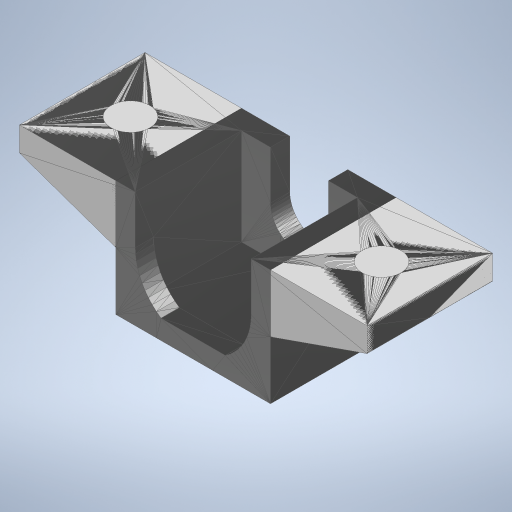
# Autodesk Inventor part: N20
Saved by Autodesk Inventor 2024 (Build 280153020, 153B)
## iProperties
Created: 2025-01-23
Part Number: N20
Material: Ogólny
Document SubType Name: Modeling
Designer: jakub
Density: 1 g/cm^3
Appearance: Domyślna
Author: jakub
Autodesk Inventor part; units mm, degrees
ref_plane "YZ Plane" through (0, 0, 0) normal (1, 0, 0) x (0, 1, 0)
ref_plane "XZ Plane" through (0, 0, 0) normal (0, 1, 0) x (-1, 0, 0)
ref_plane "XY Plane" through (0, 0, 0) normal (0, 0, 1) x (1, 0, 0)
sketch "Szkic1" plane through (78, -70, 13) normal (0, 0, 1) x (1, 0, 0)
  line L0 (-10, 0) -> (-10, -3.5)
  line L1 (-10, -3.5) -> (0, 0)
  line L2 (-10, 0) -> (-10, 2.5)
  line L3 (-10, 2.5) -> (0, 2.5)
  line L4 (0, 2.5) -> (0, 0)
  line L5 (-36, 0) -> (-36, 2.5)
  line L6 (-36, 2.5) -> (-26, 2.5)
  line L7 (-26, 2.5) -> (-26, -3.5)
  line L8 (-26, -3.5) -> (-36, 0)
  point P0 (-78, 70)
  dimension "d0" = 10
  dimension "d1" = 3.5
  dimension "d4" = 2.5
  dimension "d5" = 36
  dimension "d6" = 10
  dimension "d7" = 10
  constraints: 18 end point, 3 perpendicular, 1 horizontal, 1 vertical
  measures "d0" distance of L1.end L0.start
  measures "d1" distance of L0.start L0.end
  measures "d4" distance of L0.start L2.end
  measures "d5" distance of L1.end L5.start
  measures "d6" distance of L2.end L3.end
  measures "d7" distance of L5.end L6.end
extrude "Wyciągnięcie proste1" add sketch "Szkic1" against normal blind 13
